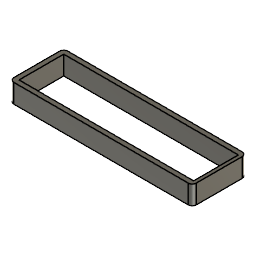
Front clock pice large (Autodesk Fusion 360 design; units mm, degrees)
part number: 2026-01-20-20-36-04-765
Autodesk Fusion 360 part; units mm, degrees
sketch "Sketch1" plane through (0, 0, 0) normal (0, 0, 1) x (1, 0, 0)
  line L0 (0, 0) -> (135, 0)
  line L1 (135, 0) -> (135, 40)
  line L2 (135, 40) -> (0, 40)
  line L3 (0, 40) -> (0, 0)
  line L4 (3.5, 36.5) -> (132.5, 36.5)
  line L5 (132.5, 36.5) -> (132.5, 3.5)
  line L6 (132.5, 3.5) -> (3.5, 3.5)
  line L7 (3.5, 3.5) -> (3.5, 36.5)
  dimension "d1" = 135
  dimension "d2" = 129
  dimension "d3" = 33
  dimension "d4" = 40
  dimension "d5" = 3.5
  dimension "d6" = 3.5
  constraint horizontal L0
  constraint vertical L1
  constraint horizontal L2
  constraint vertical L3
  constraint coincident L0.start L3.end
  constraint horizontal L4
  constraint vertical L5
  constraint horizontal L6
  constraint vertical L7
  measures "d1" distance of L0.start L0.end
  measures "d2" distance of L5.end L6.end
  measures "d3" distance of L4.start L6.end
  measures "d4" distance of L0.start L2.end
  measures "d5" distance of L2 L4
  measures "d6" distance of L3 L7
extrude "Extrude2" add sketch "Sketch1" along normal blind 14
fillet "Fillet2" radius 3 4 edges at (135, 0, 7) (135, 40, 7) (0, 0, 7) (0, 40, 7)
extrude "Extrude1" [suppressed]
fillet "Fillet1" [suppressed]
